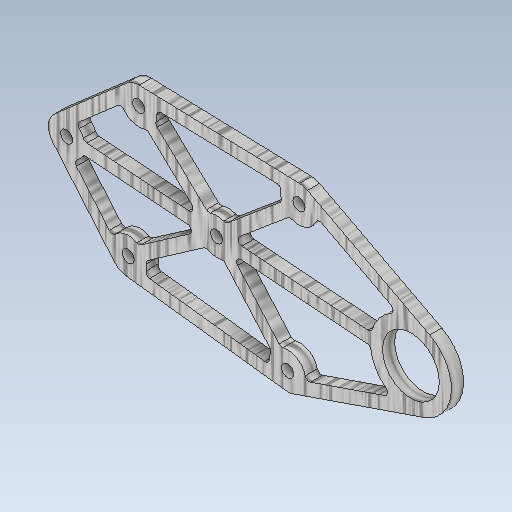
# Autodesk Inventor part: ギアトレイン
Saved by Autodesk Inventor 2020 (Build 240168000, 168)
## iProperties
Created: 2019-09-17
Part Number: ギアトレイン
Material: アルミニウム 7075
Document SubType Name: Modeling
Designer: tanjihayato
Density: 2.81 g/cm^3
Appearance: サテン - ブラシ仕上げ 重厚
Mass: 11.5797 g
Surface Area: 51.6362 cm^2
Volume: 4.12087 cm^3
Author: tanjihayato
Autodesk Inventor part; units mm, degrees
ref_plane "YZ Plane" through (0, 0, 0) normal (1, 0, 0) x (0, 1, 0)
ref_plane "XZ Plane" through (0, 0, 0) normal (0, 1, 0) x (-1, 0, 0)
ref_plane "XY Plane" through (0, 0, 0) normal (0, 0, 1) x (1, 0, 0)
sketch "スケッチ1" plane through (0, 0, 0) normal (0, 0, 1) x (1, 0, 0)
  circle A0 centre (25.3202, -9.9362) radius 19.1 construction
  circle A1 centre (62.4131, -12.7569) radius 22.1 construction
  circle A2 centre (110.4743, -16.4118) radius 30.1 construction
  circle A3 centre (25.3202, -9.9362) radius 1.5
  circle A4 centre (110.4743, -16.4118) radius 7.025
  arc A5 (22.3659, -6.5417) -> (21.8866, -12.8448) centre (25.3202, -9.9362) ccw
  arc A6 (43.2599, 10.0553) -> (40.1678, 8.9519) centre (43.1221, 5.5575) ccw
  arc A7 (37.1409, -30.8522) -> (40.0306, -32.4106) centre (40.5745, -27.9436) ccw
  arc A8 (84.879, 8.3271) -> (82.9273, 8.8396) centre (82.7895, 4.3417) ccw
  arc A9 (79.4256, -37.2072) -> (81.4324, -36.9958) centre (79.9695, -32.7402) ccw
  arc A10 (113.7333, -25.8923) -> (115.1294, -7.5331) centre (110.4743, -16.4118) ccw
  line L0 (22.3659, -6.5417) -> (40.1678, 8.9519)
  line L1 (43.2599, 10.0553) -> (82.9273, 8.8396)
  line L2 (84.879, 8.3271) -> (115.1294, -7.5331)
  line L3 (113.7333, -25.8923) -> (81.4324, -36.9958)
  line L4 (79.4256, -37.2072) -> (40.0306, -32.4106)
  line L5 (37.1409, -30.8522) -> (21.8866, -12.8448)
  circle A11 centre (62.4131, -12.7569) radius 1.5
  circle A12 centre (62.4131, -12.7569) radius 4.5 construction
  circle A13 centre (43.1221, 5.5575) radius 1.5
  circle A14 centre (82.7895, 4.3417) radius 1.5
  circle A15 centre (79.9695, -32.7402) radius 1.5
  circle A16 centre (40.5745, -27.9436) radius 1.5
  line L6 (25.3202, -9.9362) -> (102.5386, -46.4118) construction
  line L7 (25.3202, -9.9362) -> (108.6869, 8.5882) construction
  line L8 (110.4743, -16.4118) -> (33.2559, 20.0638) construction
  line L9 (110.4743, -16.4118) -> (27.1076, -34.9362) construction
  circle A17 centre (33.2559, 20.0638) radius 1.5 construction
  circle A18 centre (27.1076, -34.9362) radius 1.5 construction
  circle A19 centre (33.2559, 20.0638) radius 4.5 construction
  circle A20 centre (27.1076, -34.9362) radius 4.5 construction
  circle A21 centre (25.3202, -9.9362) radius 23.6 construction
  circle A22 centre (33.2559, 20.0638) radius 23.6 construction
  circle A23 centre (27.1076, -34.9362) radius 23.6 construction
  circle A24 centre (110.4743, -16.4118) radius 34.6 construction
  circle A25 centre (92.0329, 12.864) radius 4.5 construction
  circle A26 centre (76.1489, -20.7622) radius 4.5 construction
  line L10 (110.4743, -16.4118) -> (25.3202, -9.9362) construction
  line L11 (95.4086, 15.8397) -> (117.9946, -9.7827) construction
  line L12 (110.1305, -26.4309) -> (75.9946, -25.2595) construction
  circle A27 centre (86.0236, -40.8929) radius 4.5 construction
  line L13 (116.3452, -24.5379) -> (88.6589, -44.5405) construction
  point P0 (0, 0)
  point P1 (0, 0)
  dimension "d18" = 9
  dimension "d19" = 9
  dimension "d23" = 9
  dimension "d0" = 3
  dimension "d1" = 14.05
  dimension "d2" = 9
  dimension "d3" = 9
  dimension "d4" = 9
  dimension "d5" = 9
  dimension "d6" = 9
  dimension "d7" = 3
  dimension "d8" = 3
  dimension "d9" = 3
  dimension "d10" = 3
  dimension "d11" = 3
  dimension "d12" = 3
  dimension "d13" = 3
  dimension "d14" = 3
  dimension "d15" = 3
  dimension "d16" = 3
  dimension "d17" = 3
  dimension "d20" = 32.508
  dimension "d21" = 32.508
  dimension "d22" = 32.508
  dimension "d24" = 32.508
  constraints: 28 end point, 24 centre point, 23 tangent, 19 point on circle, 14 coincident, 2 equal length, 2 parallel, 17 other
  measures "d0" diameter of A3
  measures "d1" diameter of A4
  measures "d2" diameter of A5
  measures "d3" diameter of A6
  measures "d4" diameter of A7
  measures "d5" diameter of A8
  measures "d6" diameter of A9
  measures "d7" radial gap between concentric circles of A4 A10
  measures "d8" diameter of A11
  measures "d9" radial gap between concentric circles of A11 A12
  measures "d10" diameter of A13
  measures "d11" diameter of A14
  measures "d12" diameter of A15
  measures "d13" diameter of A16
  measures "d14" diameter of A17
  measures "d15" diameter of A18
  measures "d16" radial gap between concentric circles of A17 A19
  measures "d17" radial gap between concentric circles of A18 A20
extrude "押し出し1" add sketch "スケッチ1" along normal blind 3
sketch "スケッチ2" plane through (0, 0, 3) normal (0, 0, 1) x (1, 0, 0)
  circle A0 centre (110.4743, -16.4118) radius 7.025 projected
  circle A1 centre (40.5745, -27.9436) radius 1.5 projected
  circle A2 centre (79.9695, -32.7402) radius 1.5 projected
  circle A3 centre (82.7895, 4.3417) radius 1.5 projected
  circle A4 centre (43.1221, 5.5575) radius 1.5 projected
  circle A5 centre (62.4131, -12.7569) radius 1.5 projected
  circle A6 centre (25.3202, -9.9362) radius 1.5 projected
  arc A7 (22.3659, -6.5417) -> (21.8866, -12.8448) centre (25.3202, -9.9362) ccw projected
  line L0 (21.8866, -12.8448) -> (37.1409, -30.8522) projected
  arc A8 (37.1409, -30.8522) -> (40.0306, -32.4106) centre (40.5745, -27.9436) ccw projected
  line L1 (40.0306, -32.4106) -> (79.4256, -37.2072) projected
  arc A9 (79.4256, -37.2072) -> (81.4324, -36.9958) centre (79.9695, -32.7402) ccw projected
  line L2 (81.4324, -36.9958) -> (113.7333, -25.8923) projected
  arc A10 (113.7333, -25.8923) -> (115.1294, -7.5331) centre (110.4743, -16.4118) ccw projected
  line L3 (115.1294, -7.5331) -> (84.879, 8.3271) projected
  arc A11 (84.879, 8.3271) -> (82.9273, 8.8396) centre (82.7895, 4.3417) ccw projected
  line L4 (82.9273, 8.8396) -> (43.2599, 10.0553) projected
  arc A12 (43.2599, 10.0553) -> (40.1678, 8.9519) centre (43.1221, 5.5575) ccw projected
  line L5 (40.1678, 8.9519) -> (22.3659, -6.5417) projected
  arc A13 (38.937, 3.9036) -> (47.4087, 6.9268) centre (43.1221, 5.5575) ccw
  arc A14 (78.5948, 5.971) -> (87.2435, 3.7001) centre (82.7895, 4.3417) ccw
  arc A15 (84.4694, -32.7795) -> (75.5767, -33.7164) centre (79.9695, -32.7402) ccw
  arc A16 (44.6047, -29.9454) -> (36.6876, -25.6759) centre (40.5745, -27.9436) ccw
  arc A17 (26.918, -14.143) -> (27.5357, -6.0194) centre (25.3202, -9.9362) ccw
  circle A18 centre (62.4131, -12.7569) radius 4.5
  arc A19 (107.4023, -6.8691) -> (105.9946, -25.3802) centre (110.4743, -16.4118) ccw
  line L6 (43.168, 7.0568) -> (82.8354, 5.841)
  arc A20 (83.486, 5.6702) -> (82.8354, 5.841) centre (82.7895, 4.3417) ccw
  line L7 (83.486, 5.6702) -> (113.7364, -10.1901)
  arc A21 (112.758, -23.0552) -> (113.7364, -10.1901) centre (110.4743, -16.4118) ccw
  line L8 (112.758, -23.0552) -> (80.4572, -34.1588)
  arc A22 (79.7882, -34.2292) -> (80.4572, -34.1588) centre (79.9695, -32.7402) ccw
  line L9 (79.7882, -34.2292) -> (40.3932, -29.4326)
  arc A23 (39.4299, -28.9131) -> (40.3932, -29.4326) centre (40.5745, -27.9436) ccw
  line L10 (39.4299, -28.9131) -> (24.1757, -10.9057)
  arc A24 (24.3354, -8.8047) -> (24.1757, -10.9057) centre (25.3202, -9.9362) ccw
  line L11 (24.3354, -8.8047) -> (42.1373, 6.6889)
  arc A25 (43.168, 7.0568) -> (42.1373, 6.6889) centre (43.1221, 5.5575) ccw
  line L12 (43.1221, 5.5575) -> (62.4131, -12.7569) construction
  line L13 (42.0893, 4.4696) -> (61.3803, -13.8448)
  line L14 (63.4459, -11.6691) -> (44.1549, 6.6453)
  arc A26 (44.1549, 6.6453) -> (42.0893, 4.4696) centre (43.1221, 5.5575) ccw
  arc A27 (61.3803, -13.8448) -> (63.4459, -11.6691) centre (62.4131, -12.7569) ccw
  line L15 (82.7895, 4.3417) -> (62.4131, -12.7569) construction
  line L16 (81.8253, 5.4908) -> (61.4489, -11.6079)
  line L17 (63.3773, -13.906) -> (83.7537, 3.1927)
  arc A28 (83.7537, 3.1927) -> (81.8253, 5.4908) centre (82.7895, 4.3417) ccw
  arc A29 (61.4489, -11.6079) -> (63.3773, -13.906) centre (62.4131, -12.7569) ccw
  line L18 (79.9695, -32.7402) -> (62.4131, -12.7569) construction
  line L19 (81.0964, -31.7502) -> (63.54, -11.7669)
  line L20 (61.2862, -13.747) -> (78.8427, -33.7302)
  arc A30 (78.8427, -33.7302) -> (81.0964, -31.7502) centre (79.9695, -32.7402) ccw
  arc A31 (63.54, -11.7669) -> (61.2862, -13.747) centre (62.4131, -12.7569) ccw
  line L21 (40.5745, -27.9436) -> (62.4131, -12.7569) construction
  line L22 (41.4309, -29.1751) -> (63.2695, -13.9884)
  line L23 (61.5567, -11.5254) -> (39.7181, -26.7121)
  arc A32 (39.7181, -26.7121) -> (41.4309, -29.1751) centre (40.5745, -27.9436) ccw
  arc A33 (63.2695, -13.9884) -> (61.5567, -11.5254) centre (62.4131, -12.7569) ccw
  line L24 (25.3202, -9.9362) -> (62.4131, -12.7569) construction
  line L25 (25.2065, -11.4319) -> (62.2994, -14.2526)
  line L26 (62.5268, -11.2613) -> (25.4339, -8.4405)
  arc A34 (25.4339, -8.4405) -> (25.2065, -11.4319) centre (25.3202, -9.9362) ccw
  arc A35 (62.2994, -14.2526) -> (62.5268, -11.2613) centre (62.4131, -12.7569) ccw
  line L27 (62.4131, -12.7569) -> (110.4743, -16.4118) construction
  line L28 (62.2994, -14.2526) -> (110.3606, -17.9075)
  line L29 (110.5881, -14.9161) -> (62.5268, -11.2613)
  arc A36 (62.5268, -11.2613) -> (62.2994, -14.2526) centre (62.4131, -12.7569) ccw
  arc A37 (110.3606, -17.9075) -> (110.5881, -14.9161) centre (110.4743, -16.4118) ccw
  point P0 (0, 0)
  point P1 (52.7676, -3.5997)
  point P2 (72.6013, -4.2076)
  point P3 (71.1913, -22.7486)
  point P4 (51.4938, -20.3503)
  point P5 (43.8666, -11.3466)
  point P6 (86.4437, -14.5844)
  dimension "d27" = 3
  dimension "d28" = 3
  dimension "d29" = 3
  dimension "d30" = 3
  dimension "d31" = 3
  dimension "d32" = 3
  dimension "d33" = 3
  dimension "d34" = 3
  dimension "d35" = 3
  dimension "d36" = 3
  dimension "d37" = 3
  dimension "d38" = 3
  dimension "d39" = 3
  dimension "d40" = 3
  constraints: 60 end point, 48 point on circle, 25 centre point, 24 tangent, 12 point on line, 7 parallel, 6 coincident, 6 midpoint, 3 concentric, 11 other
  measures "d27" radial gap between concentric circles of A5 A18
  measures "d28" distance between parallel lines of L4 L6
  measures "d29" diameter of A27
  measures "d30" diameter of A29
  measures "d31" diameter of A31
  measures "d32" diameter of A33
  measures "d33" diameter of A35
  measures "d34" diameter of A37
  measures "d35" radial gap between concentric circles of A13 A4
  measures "d36" radial gap between concentric circles of A17 A6
  measures "d37" radial gap between concentric circles of A16 A1
  measures "d38" radial gap between concentric circles of A15 A2
  measures "d39" radial gap between concentric circles of A19 A0
  measures "d40" radial gap between concentric circles of A14 A3
extrude "押し出し2" cut sketch "スケッチ2" against normal blind 10 contours A19 L29 A18 L17 A14 L7 | L8 A15 L19 A18 L28 A19 | A19 L28 A18 L29 | L17 A18 L16 A14 | A15 L20 A18 L19 | L16 A18 L14 A13 L6 A14 | A15 L9 A16 L22 A18 L20 | A18 L13 A13 L14 | L22 A16 L23 A18 | A18 L26 A17 L11 A13 L13 | L23 A16 L10 A17 L25 A18 | A18 L25 A17 L26
extrude "押し出し3" add sketch "スケッチ2" against normal blind 3 contours L29 A37 L28 A0 | A0 L28 A19 L29 | A19 L28 A18 L29 | A18 L28 L19 L17 L29 | L17 A18 L16 A14 | A14 L16 A3 L17 | L19 A2 L20 A15 | A15 L20 A18 L19 | L17 L29 L14 L16 A18 | L17 L19 A5 L14 L29 | A18 L20 L22 L28 L19 | L28 L22 A5 L17 L19 | L17 A5 L19 | L29 L26 L16 L14 | L14 A5 L29 | L28 A5 L22 | L22 L20 L25 L28 | L14 L16 L26 L13 A18 | A18 L13 A13 L14 | A5 L16 L26 | L22 A16 L23 A18 | A18 L23 L25 L20 L22 | L25 L20 A5 | A13 L13 A4 L14 | L16 L23 L13 L26 | L22 A1 L23 A16 | L25 L23 L13 L20 | L26 L13 L23 L25 A18 | A18 L25 A17 L26 | A5 L13 L23 | A17 L25 A6 L26 picked at (108.1581, -16.0674)
extrude "押し出し4" cut sketch "スケッチ2" against normal blind 3 contours A0 L28 A37 L29 | L29 A37 L28 A0
fillet "フィレット1" radius 1 36 edges at (44.6047, -29.9454, 1.5) (44.9141, -26.7529, 1.5) (75.5767, -33.7164, 1.5) (59.7863, -16.4107, 1.5) (76.0424, -30.543, 1.5) (64.0864, -16.9343, 1.5) (26.918, -14.143, 1.5) (29.4369, -11.7536, 1.5) (36.6876, -25.6759, 1.5) (58.0689, -13.9309, 1.5) (43.2013, -24.2899, 1.5) (58.0735, -13.9477, 1.5) (84.4694, -32.7795, 1.5) (78.2962, -28.5629, 1.5) (105.9946, -25.3802, 1.5) (66.3402, -14.9542, 1.5) (100.477, -17.1559, 1.5) (66.5298, -14.5743, 1.5) (38.937, 3.9036, 1.5) (45.1662, 1.5485, 1.5) (27.5357, -6.0194, 1.5) (58.3035, -10.9237, 1.5) (29.6644, -8.7622, 1.5) (58.2964, -10.9396, 1.5) (78.5948, 5.971, 1.5) (78.5753, 2.7636, 1.5) (47.4087, 6.9268, 1.5) (64.6989, -8.8807, 1.5) (47.2317, 3.7242, 1.5) (60.369, -8.748, 1.5) (107.4023, -6.8691, 1.5) (100.7045, -14.1645, 1.5) (87.2435, 3.7001, 1.5) (66.7573, -11.583, 1.5) (80.5037, 0.4655, 1.5) (66.6273, -11.1788, 1.5)
equation "\"d21\" = d20"
equation "\"d22\" = d20"
equation "\"d24\" = d20"
